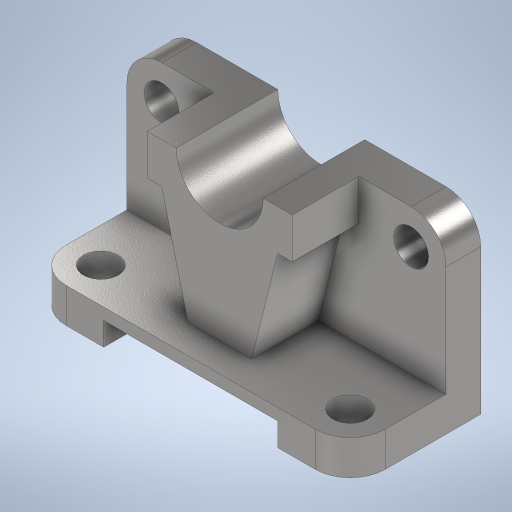
# Autodesk Inventor part: manu
Saved by Autodesk Inventor 2024 (Build 280153000, 153)
## iProperties
Created: 2024-02-01
Part Number: manu
Material: Stahl, galvanisiert
Document SubType Name: Modeling
Designer: ffogue
Density: 7.85 g/cm^3
Appearance: Galvanisiert
Author: ffogue
Autodesk Inventor part; units mm, degrees
ref_plane "YZ Plane" through (0, 0, 0) normal (1, 0, 0) x (0, 1, 0)
ref_plane "XZ Plane" through (0, 0, 0) normal (0, 1, 0) x (-1, 0, 0)
sketch "Skizze1" plane through (0, 0, 0) normal (0, 0, 1) x (1, 0, 0)
  line L0 (0, 45) -> (110, 45)
  line L1 (110, 45) -> (110, 0)
  line L2 (110, 0) -> (0, 0)
  line L3 (0, 0) -> (0, 45)
  dimension "d0" = 110
  dimension "d1" = 45
  constraints: 8 end point, 2 parallel, 1 coincident, 1 horizontal, 1 perpendicular
  measures "d0" distance between parallel lines of L1 L3
  measures "d1" distance between parallel lines of L2 L0
extrude "Extrusion1" add sketch "Skizze1" along normal blind 12
sketch "Skizze2" plane through (110, 0, 0) normal (1, 0, 0) x (0, 0, -1)
  line L0 (0, 45) -> (-12, 45) projected
  line L1 (0, 45) -> (-62, 45)
  line L2 (-62, 45) -> (-62, 33)
  line L3 (-62, 33) -> (0, 33)
  line L4 (0, 33) -> (0, 45)
  point P0 (0, 0)
  dimension "d4" = 12
  dimension "d5" = 62
  constraints: 8 end point, 2 parallel, 1 horizontal, 1 perpendicular
  measures "d4" distance between parallel lines of L3 L1
  measures "d5" distance between parallel lines of L2 L4
extrude "Extrusion2" add sketch "Skizze2" against normal up to surface (110 mm away)
fillet "Rundung1" radius 12 4 edges at (110, 0, 6) (0, 0, 6) (0, 39, 62) (110, 39, 62)
ref_plane "Arbeitsebene1" through (0, 0, 48) normal (0, 0, 1) x (1, 0, 0)
sketch "Skizze5" plane through (0, 0, 48) normal (0, 0, 1) x (1, 0, 0)
  line L0 (110, 45) -> (0, 45) projected
  line L1 (30, 45) -> (80, 45)
  line L2 (80, 45) -> (80, 10)
  line L3 (80, 10) -> (30, 10)
  line L4 (30, 10) -> (30, 45)
  line L5 (12, 0) -> (98, 0) projected
  point P0 (0, 0)
  point P1 (55, 10)
  point P2 (55, 0)
  dimension "d12" = 50
  dimension "d13" = 35
  constraints: 8 end point, 2 midpoint, 2 parallel, 1 horizontal, 1 perpendicular, 1 point on line, 1 vertical alignment
  measures "d12" distance of L2.end L3.end
  measures "d13" distance of L1.end L2.end
extrude "Extrusion4" add sketch "Skizze5" along normal up to surface (14 mm away)
sketch "Skizze3" plane through (0, 0, 12) normal (0, 0, 1) x (1, 0, 0)
  line L0 (98, 33) -> (12, 33) projected
  line L1 (44, 33) -> (66, 33)
  line L2 (66, 33) -> (66, 10)
  line L3 (66, 10) -> (44, 10)
  line L4 (44, 10) -> (44, 33)
  line L5 (12, 0) -> (98, 0) projected
  point P0 (0, 0)
  point P1 (55, 10)
  point P2 (55, 0)
  dimension "d9" = 22
  dimension "d10" = 23
  constraints: 8 end point, 2 midpoint, 2 parallel, 1 horizontal, 1 perpendicular, 1 point on line, 1 vertical alignment
  measures "d9" distance of L2.end L3.end
  measures "d10" distance of L1.end L2.end
sketch "Skizze9" plane through (0, 0, 48) normal (0, 0, -1) x (-1, 0, 0)
  line L0 (-80, 10) -> (-30, 10) projected
  line L1 (-35, 33) -> (-75, 33)
  line L2 (-75, 33) -> (-75, 10)
  line L3 (-75, 10) -> (-35, 10)
  line L4 (-35, 10) -> (-35, 33)
  line L5 (-98, 45) -> (-12, 45) projected
  point P0 (0, 0)
  point P1 (-55, 33)
  point P2 (-55, 45)
  dimension "d30" = 40
  dimension "d31" = 23
  constraints: 8 end point, 2 midpoint, 2 parallel, 1 horizontal, 1 perpendicular, 1 point on line, 1 vertical alignment
  measures "d30" distance between parallel lines of L2 L4
  measures "d31" distance between parallel lines of L1 L0
loft "Erhebung3" add profiles "Skizze3", "Skizze9"
sketch "Skizze10" plane through (30, 10, 62) normal (0, -1, 0) x (1, 0, 0)
  line L0 (68, 0) -> (-18, 0) projected
  arc A0 (10, 0) -> (40, 0) centre (25, 0) ccw
  line L1 (0, -14) -> (0, 0) projected
  line L2 (50, -14) -> (50, 0) projected
  point P0 (-30, -62)
  dimension "d38" = 30
  dimension "d39" = 10
  constraints: 2 point on circle, 2 point on line, 1 centre point, 1 midpoint
  measures "d38" distance of A0.end A0.start
  measures "d39" distance from line of L1 A0.start
extrude "Extrusion5" cut sketch "Skizze10" against normal up to surface (35 mm away)
sketch "Skizze11" plane through (0, 33, 12) normal (0, -1, 0) x (1, 0, 0)
  arc A0 (12, 50) -> (0, 38) centre (12, 38) ccw projected
  point P0 (0, -12)
  constraints: 1 coincident
hole "Bohrung1" at (12, 33, 50) direction (0, 1, 0) diameter 12 depth 12
sketch "Skizze12" plane through (110, 33, 12) normal (0, -1, 0) x (1, 0, 0)
  arc A0 (0, 38) -> (-12, 50) centre (-12, 38) ccw projected
  point P0 (-110, -12)
  constraints: 1 coincident
hole "Bohrung2" at (98, 33, 50) direction (0, 1, 0) diameter 12 depth 12
sketch "Skizze13" plane through (0, 0, 12) normal (0, 0, 1) x (1, 0, 0)
  arc A0 (98, 0) -> (110, 12) centre (98, 12) ccw projected
  point P0 (0, 0)
  constraints: 1 coincident
hole "Bohrung3" at (98, 12, 12) direction (0, 0, -1) diameter 12 depth 12
sketch "Skizze14" plane through (0, 0, 12) normal (0, 0, 1) x (1, 0, 0)
  arc A0 (0, 12) -> (12, 0) centre (12, 12) ccw projected
  point P0 (0, 0)
  constraints: 1 coincident
hole "Bohrung4" at (12, 12, 12) direction (0, 0, -1) diameter 12 depth 12
sketch "Skizze15" plane through (12, 0, 0) normal (0, -1, 0) x (1, 0, 0)
  line L0 (0, 0) -> (86, 0) projected
  line L1 (13, 0) -> (73, 0)
  line L2 (73, 0) -> (73, 8)
  line L3 (73, 8) -> (13, 8)
  line L4 (13, 8) -> (13, 0)
  line L5 (-12, 12) -> (-12, 0) projected
  dimension "d70" = 60
  dimension "d71" = 25
  dimension "d72" = 8
  constraints: 8 end point, 2 parallel, 1 horizontal, 1 perpendicular, 1 point on line
  measures "d70" distance between parallel lines of L2 L4
  measures "d71" distance between parallel lines of L5 L4
  measures "d72" distance between parallel lines of L0 L3
extrude "Extrusion6" cut sketch "Skizze15" against normal up to surface (45 mm away)
